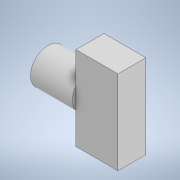
# Autodesk Inventor part: Gripper
Saved by Autodesk Inventor 2020 (Build 240168000, 168)
## iProperties
Created: 2020-12-23
Part Number: Gripper
Material: Generic
Document SubType Name: Modeling
Designer: frost
Density: 1 g/cm^3
Appearance: Default
Author: frost
Autodesk Inventor part; units mm, degrees
ref_plane "YZ Plane" through (0, 0, 0) normal (1, 0, 0) x (0, 1, 0)
ref_plane "XZ Plane" through (0, 0, 0) normal (0, 1, 0) x (-1, 0, 0)
ref_plane "XY Plane" through (0, 0, 0) normal (0, 0, 1) x (1, 0, 0)
sketch "Sketch1" plane through (0, 0, 0) normal (1, 0, 0) x (0, 1, 0)
  circle A0 centre (0, 0) radius 2.5
  dimension "d0" = 5
  constraints: 1 centre point, 1 coincident
  measures "d0" diameter of A0
extrude "Extrusion1" add sketch "Sketch1" along normal blind 6
sketch "Sketch2" plane through (6, 0, 0) normal (1, 0, 0) x (0, 0, -1)
  line L0 (-2, 6) -> (2, 6)
  line L1 (2, 6) -> (2, -6)
  line L2 (2, -6) -> (-2, -6)
  line L3 (-2, -6) -> (-2, 6)
  line L4 (-2, 6) -> (2, -6) construction
  line L5 (2, 6) -> (-2, -6) construction
  point P0 (0, 0)
  dimension "d3" = 4
  dimension "d4" = 12
  constraints: 12 end point, 2 midpoint, 2 parallel, 1 horizontal, 1 perpendicular
  measures "d3" distance of L1.end L2.end
  measures "d4" distance of L0.end L1.end
extrude "Extrusion2" add sketch "Sketch2" along normal blind 6
sketch "Sketch3" plane through (6, 1.5, 2) normal (0, 0, 1) x (1, 0, 0)
  point P0 (-6, -1.5)
body "Solid1"
